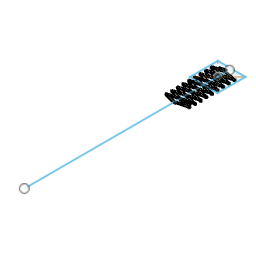
Scissor Cable Management_ (Autodesk Fusion 360 design; units mm, degrees)
Autodesk Fusion 360 part; units mm, degrees
sketch "Sketch1" plane through (0, 0, 0) normal (0, 1, 0) x (1, 0, 0) in component "Bottom"
  line L0 (0, 0) -> (0, 9) construction
  line L1 (0, 0) -> (54.8156, 4.5) construction
  line L2 (54.8156, 4.5) -> (0, 9) construction
  line L3 (0, 4.5) -> (54.8156, 4.5) construction
  line L4 (0, 9) -> (-54.8156, 13.5) construction
  line L5 (0, 0) -> (-54.8156, -4.5) construction
  line L6 (-55.1429, 9.5134) -> (54.4883, 0.5134)
  arc A0 (54.4883, 0.5134) -> (55.1429, 8.4866) centre (54.8156, 4.5) ccw
  line L7 (55.1429, 8.4866) -> (-54.4883, 17.4866)
  arc A1 (-54.4883, 17.4866) -> (-55.1429, 9.5134) centre (-54.8156, 13.5) ccw
  line L8 (-54.8156, 13.5) -> (54.8156, 4.5) construction
  line L9 (54.4883, 8.4866) -> (-55.1429, -0.5134)
  arc A2 (-55.1429, -0.5134) -> (-54.4883, -8.4866) centre (-54.8156, -4.5) ccw
  line L10 (-54.4883, -8.4866) -> (55.1429, 0.5134)
  arc A3 (55.1429, 0.5134) -> (54.4883, 8.4866) centre (54.8156, 4.5) ccw
  line L11 (54.8156, 4.5) -> (-54.8156, -4.5) construction
  circle A4 centre (-54.8156, -4.5) radius 1.6
  circle A5 centre (54.8156, 4.5) radius 1.6
  circle A6 centre (-54.8156, 13.5) radius 1.6
  circle A7 centre (0, 9) radius 1.6
  circle A8 centre (0, 0) radius 1.6
  circle A9 centre (0, 9) radius 4.5 construction
  circle A10 centre (0, 0) radius 4.5 construction
  point P0 (0, 4.5)
  dimension "d5" = 55
  dimension "d8" = 55
  dimension "d10" = 55
  dimension "d11" = 8
  dimension "d12" = 8
  dimension "d13" = 3.2
  dimension "d14" = 3.2
  dimension "d15" = 3.2
  dimension "d16" = 3.2
  dimension "d17" = 3.2
  dimension "d18" = 9
  dimension "d19" = 9
  constraint coincident L0.start L1.start
  constraint vertical L0
  constraint midpoint L0 P0
  constraint coincident P0 L3.start
  constraint horizontal L3
  constraint parallel L2 L4
  constraint parallel L1 L5
  constraint tangent L6 A0
  constraint tangent A0 L7
  constraint parallel L6 L7
  constraint tangent L7 A1
  constraint tangent L6 A1
  constraint coincident L1.end L2.start
  constraint parallel L2 L8
  constraint coincident L4.end A1.centre
  constraint tangent L9 A2
  constraint tangent A2 L10
  constraint parallel L9 L10
  constraint tangent L10 A3
  constraint tangent L9 A3
  constraint coincident L5.end A2.centre
  constraint parallel L5 L11
  constraint concentric A2 A4
  constraint concentric A3 A5
  constraint concentric A1 A6
  constraint coincident L0.end L2.end
  constraint concentric A7 A9
  constraint tangent A9 A10
  measures "d5" distance of L0.start L1.end
  measures "d8" distance of L0.end L4.end
  measures "d10" distance of L0.start L5.end
  measures "d11" diameter of A0
  measures "d12" diameter of A2
  measures "d13" diameter of A4
  measures "d14" diameter of A5
  measures "d15" diameter of A6
  measures "d16" diameter of A7
  measures "d17" diameter of A8
  measures "d18" diameter of A9
  measures "d19" diameter of A10
extrude "Extrude1" add sketch "Sketch1" along normal blind 3 contours L6 L7 A1 L9 A3 | L6 A0 L9 A3 makes body 1 in component "1"
extrude "Extrude1'" add sketch "Sketch1" against normal blind 3 separate body contours L6 A0 L9 A3 | L6 A0 L9 A2 L10 makes body 2 in component "2"
pattern_linear "00000000-0000-0000-0000-000000000000" [suppressed] in component "Bottom"
sketch "Sketch1 (2)" plane through (0, 0, 0) normal (0, 1, 0) x (1, 0, 0) in component "Top"
  line L0 (0, 0) -> (0, 9) construction
  line L1 (0, 0) -> (54.8156, 4.5) construction
  line L2 (54.8156, 4.5) -> (0, 9) construction
  line L3 (0, 4.5) -> (54.8156, 4.5) construction
  line L4 (0, 9) -> (-54.8156, 13.5) construction
  line L5 (0, 0) -> (-54.8156, -4.5) construction
  line L6 (-55.1429, 9.5134) -> (54.4883, 0.5134)
  arc A0 (54.4883, 0.5134) -> (55.1429, 8.4866) centre (54.8156, 4.5) ccw
  line L7 (55.1429, 8.4866) -> (-54.4883, 17.4866)
  arc A1 (-54.4883, 17.4866) -> (-55.1429, 9.5134) centre (-54.8156, 13.5) ccw
  line L8 (-54.8156, 13.5) -> (54.8156, 4.5) construction
  line L9 (54.4883, 8.4866) -> (-55.1429, -0.5134)
  arc A2 (-55.1429, -0.5134) -> (-54.4883, -8.4866) centre (-54.8156, -4.5) ccw
  line L10 (-54.4883, -8.4866) -> (55.1429, 0.5134)
  arc A3 (55.1429, 0.5134) -> (54.4883, 8.4866) centre (54.8156, 4.5) ccw
  line L11 (54.8156, 4.5) -> (-54.8156, -4.5) construction
  circle A4 centre (-54.8156, -4.5) radius 2.15
  circle A5 centre (54.8156, 4.5) radius 2.15
  circle A6 centre (-54.8156, 13.5) radius 2.15
  circle A7 centre (0, 9) radius 2.15
  circle A8 centre (0, 0) radius 2.15
  circle A9 centre (0, 9) radius 4.5 construction
  circle A10 centre (0, 0) radius 4.5 construction
  point P0 (0, 4.5)
  dimension "d5_1" = 55
  dimension "d8_1" = 55
  dimension "d10_1" = 55
  dimension "d11_1" = 8
  dimension "d12_1" = 8
  dimension "d13_1" = 4.3
  dimension "d14_1" = 4.3
  dimension "d15_1" = 4.3
  dimension "d16_1" = 4.3
  dimension "d17_1" = 4.3
  dimension "d18_1" = 9
  dimension "d19_1" = 9
  constraint coincident L0.start L1.start
  constraint vertical L0
  constraint midpoint L0 P0
  constraint coincident P0 L3.start
  constraint horizontal L3
  constraint parallel L2 L4
  constraint parallel L1 L5
  constraint tangent L6 A0
  constraint tangent A0 L7
  constraint parallel L6 L7
  constraint tangent L7 A1
  constraint tangent L6 A1
  constraint coincident L1.end L2.start
  constraint parallel L2 L8
  constraint coincident L4.end A1.centre
  constraint tangent L9 A2
  constraint tangent A2 L10
  constraint parallel L9 L10
  constraint tangent L10 A3
  constraint tangent L9 A3
  constraint coincident L5.end A2.centre
  constraint parallel L5 L11
  constraint concentric A2 A4
  constraint concentric A3 A5
  constraint concentric A1 A6
  constraint coincident L0.end L2.end
  constraint concentric A7 A9
  constraint tangent A9 A10
  measures "d5_1" distance of L0.start L1.end
  measures "d8_1" distance of L0.end L4.end
  measures "d10_1" distance of L0.start L5.end
  measures "d11_1" diameter of A0
  measures "d12_1" diameter of A2
  measures "d13_1" diameter of A4
  measures "d14_1" diameter of A5
  measures "d15_1" diameter of A6
  measures "d16_1" diameter of A7
  measures "d17_1" diameter of A8
  measures "d18_1" diameter of A9
  measures "d19_1" diameter of A10
extrude "Extrude1''" add sketch "Sketch1 (2)" along normal blind 3 separate body contours L6 L7 A1 L9 A3 | L6 A0 L9 A3 makes body 3 in component "1 (1)"
extrude "Extrude1'''" add sketch "Sketch1 (2)" against normal blind 3 separate body contours L6 A0 L9 A3 | L6 A0 L9 A2 L10 makes body 4 in component "2 (1)"
pattern_linear "R-Pattern1" [suppressed] in component "Top"
sketch "Sketch15" plane through (0, 0, 0) normal (0, 1, 0) x (1, 0, 0)
  line L0 (65, -95.4189) -> (-65, -95.4189)
  line L1 (-65, -95.4189) -> (-65, 35.4189)
  line L2 (-65, 35.4189) -> (65, 35.4189)
  line L3 (65, 35.4189) -> (65, -95.4189)
  line L4 (65, -95.4189) -> (-65, 35.4189) construction
  line L5 (-65, -95.4189) -> (65, 35.4189) construction
  point P0 (0, -30)
  dimension "d422" = 130
  constraint horizontal L0
  constraint perpendicular L0 L1
  constraint parallel L0 L2
  constraint parallel L1 L3
  constraint coincident L4 P0
  constraint coincident L5 P0
  measures "d422" distance of L1.end L2.end
sketch "Sketch1 (3)" plane through (0, -3, 0) normal (0, -1, 0) x (1, 0, 0) in component "Adapter"
  circle A0 centre (-54.8156, -4.5) radius 1.6
  circle A1 centre (0, -9) radius 1.6
  circle A2 centre (54.8156, -13.5) radius 1.6
  arc A3 (-54.4883, -0.5134) -> (-55.1429, -8.4866) centre (-54.8156, -4.5) ccw
  line L0 (-55.1429, -8.4866) -> (54.4883, -17.4866)
  arc A4 (54.4883, -17.4866) -> (55.1429, -9.5134) centre (54.8156, -13.5) ccw
  line L1 (55.1429, -9.5134) -> (-54.4883, -0.5134)
  circle A5 centre (0, -9) radius 1.6
  line L2 (9.1446, -15.4098) -> (-9.1446, -15.4098)
  line L3 (-9.1446, -15.4098) -> (-9.1446, -2.5902)
  line L4 (-9.1446, -2.5902) -> (9.1446, -2.5902)
  line L5 (9.1446, -2.5902) -> (9.1446, -15.4098)
  line L6 (9.1446, -15.4098) -> (-9.1446, -2.5902) construction
  line L7 (-9.1446, -15.4098) -> (9.1446, -2.5902) construction
  point P0 (0, -9)
  constraint horizontal L2
  constraint perpendicular L2 L3
  constraint parallel L2 L4
  constraint parallel L3 L5
  constraint coincident L6 P0
  constraint coincident L7 P0
  constraint coincident P0 A1.centre
extrude "Extrude1''''" add sketch "Sketch1 (3)" along normal blind 4 separate body contours L1 L3 L4 L5 | L0 L1 L3 L5 | L0 L2 L3 L5 makes body 5 in component "Adapter"
sketch "Sketch4" plane through (0, 0, 0) normal (0, 1, 0) x (1, 0, 0)
  line L0 (0, 25) -> (0, -935)
  dimension "d193" = 960
  constraint vertical L0
  measures "d193" distance of L0.start L0.end
sketch "Sketch3" plane through (0, 3, 0) normal (0, 1, 0) x (-1, 0, 0) in component "Top"
  circle A0 centre (0, -9) radius 2.15
  circle A1 centre (54.2857, -0.1646) radius 2.15
  circle A2 centre (-54.2857, -17.8354) radius 2.15
  arc A3 (54.9283, -4.1127) -> (53.6431, 3.7834) centre (54.2857, -0.1646) ccw
  line L0 (53.6431, 3.7834) -> (-54.9283, -13.8873)
  arc A4 (-54.9283, -13.8873) -> (-53.6431, -21.7834) centre (-54.2857, -17.8354) ccw
  line L1 (-53.6431, -21.7834) -> (54.9283, -4.1127)
  line L2 (-54.2857, -17.8354) -> (0, -9) construction
  line L3 (0, -9) -> (54.2857, -0.1646) construction
  line L4 (-27.1428, -13.4177) -> (-27.7854, -9.4696)
  line L5 (-27.1428, -13.4177) -> (-26.5003, -17.3657) construction
  line L6 (0, -9) -> (-0.5388, -5.6896) construction
  line L7 (-24.1818, -12.9358) -> (-24.8244, -8.9877)
  line L8 (-24.1818, -12.9358) -> (-23.5392, -16.8838)
  line L9 (-30.1039, -13.8996) -> (-30.7465, -9.9516)
  line L10 (-30.1039, -13.8996) -> (-29.4613, -17.8477)
  line L11 (24.1818, -5.0642) -> (23.5392, -1.1162)
  line L12 (24.1818, -5.0642) -> (24.8244, -9.0123)
  line L13 (30.1039, -4.1004) -> (29.4613, -0.1523)
  line L14 (30.1039, -4.1004) -> (30.7465, -8.0484)
  dimension "d243" = 3
  dimension "d244" = -3
  constraint coincident A2.centre A4.centre
  constraint coincident A0.centre L2.end
  constraint coincident A1.centre A3.centre
  constraint midpoint L2 L4.start
  constraint coincident L0 L4.end
  constraint perpendicular L0 L4
  constraint coincident L1 L5.end
  constraint perpendicular L1 L5
  constraint perpendicular L3 L6
  constraint symmetric L6 L7.start L11.start
  constraint symmetric L6 L7.end L11.end
  constraint symmetric L6 L8.end L12.end
  constraint symmetric L6 L9.start L13.start
  constraint symmetric L6 L9.end L13.end
  constraint symmetric L6 L10.end L14.end
extrude "Extrude4" add sketch "Sketch3" along normal blind 6 contours L0 L1 L11 L12 L13 L14 | L0 L1 L7 L8 L9 L10 sketch seen with x (-0.97056, 0, -0.24086) y (0, 1, 0) z (0.24086, 0, -0.97056) at (2.1677, 0, -17.735) bodies 3 in component "1 (1)"
sketch "Sketch1 (4)" plane through (29.6638, 0, 2.4352) normal (0.996647, 0, 0.081818) x (0.081818, 0, -0.996647) in component "1 (1)"
  line L0 (4.9698, 3) -> (12.9698, 3)
  line L1 (12.9698, 3) -> (12.9698, 9)
  line L2 (12.9698, 9) -> (4.9698, 9)
  line L3 (4.9698, 9) -> (4.9698, 3)
  line L4 (8.9698, 9) -> (8.9698, 3) construction
  circle A0 centre (8.9698, 5) radius 4
  circle A1 centre (8.9698, 5) radius 2
  dimension "d248" = 8
  dimension "d249" = 4
  constraint midpoint L2 L4.start
  constraint midpoint L0 L4.end
  constraint coincident L4.start A0
  constraint concentric A0 A1
  measures "d248" diameter of A0
  measures "d249" diameter of A1
extrude "Extrude5" cut sketch "Sketch1 (4)" against normal blind 69 contours A1 | L2 L3 A0 | L1 L2 A0 bodies 3 in component "1 (1)"
sketch "Sketch2" plane through (0, 3, 2.4175) normal (0, 1, 0) x (-1, 0, 0) in component "Bottom"
  circle A0 centre (-54.2857, -2.5821) radius 1.6
  circle A1 centre (0, 6.2532) radius 1.6
  circle A2 centre (54.2857, 15.0886) radius 1.6
  arc A3 (-54.9283, 1.3659) -> (-53.6431, -6.5302) centre (-54.2857, -2.5821) ccw
  line L0 (-53.6431, -6.5302) -> (54.9283, 11.1406)
  arc A4 (54.9283, 11.1406) -> (53.6431, 19.0367) centre (54.2857, 15.0886) ccw
  line L1 (53.6431, 19.0367) -> (-54.9283, 1.3659)
  line L2 (0, 6.2532) -> (-54.2857, -2.5821) construction
  line L3 (0, 6.2532) -> (54.2857, 15.0886) construction
  line L4 (-27.1428, 1.8355) -> (-27.7854, 5.7836)
  line L5 (-27.1428, 1.8355) -> (-26.5003, -2.1125) construction
  line L6 (-24.1818, 2.3175) -> (-24.8244, 6.2655)
  line L7 (-24.1818, 2.3175) -> (-23.5392, -1.6306)
  line L8 (-30.1039, 1.3536) -> (-30.7465, 5.3017)
  line L9 (-30.1039, 1.3536) -> (-29.4613, -2.5944)
  line L10 (0, 6.2532) -> (-0.257, 7.8325) construction
  line L11 (24.1818, 10.189) -> (23.5392, 14.137)
  line L12 (30.1039, 11.1528) -> (29.4613, 15.1009)
  line L13 (30.1039, 11.1528) -> (30.7465, 7.2048)
  line L14 (24.1818, 10.189) -> (24.8244, 6.2409)
  dimension "d252" = 3
  dimension "d253" = -3
  constraint coincident A1.centre L2.start
  constraint coincident A0.centre A3.centre
  constraint coincident A2.centre A4.centre
  constraint midpoint L2 L4.start
  constraint coincident L1 L4.end
  constraint perpendicular L1 L4
  constraint coincident L0 L5.end
  constraint perpendicular L0 L5
  constraint coincident A1 L10.end
  constraint perpendicular L3 L10
  constraint symmetric L6.start L10 L11.start
  constraint symmetric L6.end L10 L11.end
  constraint symmetric L7.end L10 L14.end
  constraint symmetric L8.start L10 L12.start
  constraint symmetric L8.end L10 L12.end
  constraint symmetric L9.end L10 L13.end
extrude "Extrude2" add sketch "Sketch2" along normal blind 6 contours L0 L1 L6 L7 L8 L9 | L0 L1 L11 L12 L13 L14 sketch seen with x (0.97056, 0, -0.24086) y (0, -1, 0) z (-0.24086, 0, -0.97056) at (2.0884, 0, 8.4155) bodies 2 in component "2"
sketch "Sketch1 (5)" plane through (-30.3977, 0, 2.4955) normal (-0.996647, 0, 0.081818) x (0.081818, 0, 0.996647) in component "2"
  line L0 (4, -3) -> (-4, -3)
  line L1 (-4, -3) -> (-4, -9)
  line L2 (-4, -9) -> (4, -9)
  line L3 (4, -9) -> (4, -3)
  line L4 (0, -9) -> (0, -1) construction
  circle A0 centre (0, -5) radius 4
  circle A1 centre (0, -5) radius 2
  dimension "d256" = 8
  dimension "d257" = 8
  dimension "d258" = 4
  constraint midpoint L2 L4.start
  constraint perpendicular L2 L4
  constraint midpoint L4 A0.centre
  constraint concentric A0 A1
  measures "d256" distance of L4.start L4.end
  measures "d257" diameter of A0
  measures "d258" diameter of A1
extrude "Extrude3" cut sketch "Sketch1 (5)" against normal blind 68 contours A1 | L2 L3 A0 | L1 L2 A0 bodies 2 in component "2"
extrude "Extrude1'''''" add sketch "Sketch1" against normal blind 3 separate body contours L6 L7 A1 L9 A3 | L6 A0 L9 A3 makes body 6 in component "Terminator"
sketch "Sketch1 (6)" plane through (0, 0, 0) normal (0, 1, 0) x (-1, 0, 0) in component "Terminator"
  circle A0 centre (0, -9) radius 1.6
  circle A1 centre (-54.8156, -4.5) radius 1.6
  circle A2 centre (54.8156, -13.5) radius 1.6
  arc A3 (-54.4883, -0.5134) -> (-55.1429, -8.4866) centre (-54.8156, -4.5) ccw
  line L0 (-55.1429, -8.4866) -> (54.4883, -17.4866)
  arc A4 (54.4883, -17.4866) -> (55.1429, -9.5134) centre (54.8156, -13.5) ccw
  line L1 (55.1429, -9.5134) -> (-54.4883, -0.5134)
  line L2 (-55.1586, -8.6783) -> (-0.343, -13.1783)
  arc A5 (-0.343, -13.1783) -> (0.343, -4.8217) centre (0, -9) ccw
  line L3 (0.343, -4.8217) -> (-54.4726, -0.3217)
  arc A6 (-54.4726, -0.3217) -> (-55.1586, -8.6783) centre (-54.8156, -4.5) ccw
  line L4 (-54.8156, -4.5) -> (0, -9) construction
  constraint tangent L2 A5
  constraint tangent A5 L3
  constraint parallel L2 L3
  constraint tangent L3 A6
  constraint tangent L2 A6
  constraint coincident A0.centre A5.centre
  constraint parallel L0 L4
  constraint coincident A1.centre A3.centre
extrude "Extrude2'" cut sketch "Sketch1 (6)" against normal blind 3 contours L0 A4 L1 A5 bodies 6 in component "Terminator"
extrude "Extrude1''''''" add sketch "Sketch1" along normal blind 3 separate body contours L6 L7 A1 L9 A3 | L6 A0 L9 A3 makes body 7 in component "Terminator (1)"
sketch "Sketch1 (7)" plane through (0, 3, 0) normal (0, 1, 0) x (-1, 0, 0) in component "Terminator (1)"
  circle A0 centre (0, -9) radius 1.6
  circle A1 centre (-54.8156, -4.5) radius 1.6
  circle A2 centre (54.8156, -13.5) radius 1.6
  arc A3 (-54.4883, -0.5134) -> (-55.1429, -8.4866) centre (-54.8156, -4.5) ccw
  line L0 (-55.1429, -8.4866) -> (54.4883, -17.4866)
  arc A4 (54.4883, -17.4866) -> (55.1429, -9.5134) centre (54.8156, -13.5) ccw
  line L1 (55.1429, -9.5134) -> (-54.4883, -0.5134)
  line L2 (-0.343, -13.1783) -> (54.4726, -17.6783)
  arc A5 (54.4726, -17.6783) -> (55.1586, -9.3217) centre (54.8156, -13.5) ccw
  line L3 (55.1586, -9.3217) -> (0.343, -4.8217)
  arc A6 (0.343, -4.8217) -> (-0.343, -13.1783) centre (0, -9) ccw
  line L4 (0, -9) -> (54.8156, -13.5) construction
  constraint tangent L2 A5
  constraint tangent A5 L3
  constraint parallel L2 L3
  constraint tangent L3 A6
  constraint tangent L2 A6
  constraint coincident A2.centre A4.centre
  constraint coincident A0.centre A6.centre
extrude "Extrude2''" cut sketch "Sketch1 (7)" against normal blind 3 contours A3 L0 L1 A6 bodies 7 in component "Terminator (1)"
sketch "Sketch2 (2)" plane through (0, 3, 0) normal (0, 1, 0) x (-1, 0, 0) in component "Terminator (1)"
  arc A0 (-0.924, -4.9107) -> (-1.5786, -12.8839) centre (0, -9) ccw
  line L0 (-1.5786, -12.8839) -> (54.4883, -17.4866)
  arc A1 (54.4883, -17.4866) -> (55.1429, -9.5134) centre (54.8156, -13.5) ccw
  line L1 (55.1429, -9.5134) -> (-0.924, -4.9107)
  circle A2 centre (0, -9) radius 1.6
  circle A3 centre (54.8156, -13.5) radius 1.6
  line L2 (0, -9) -> (54.8156, -13.5) construction
  line L3 (27.4078, -11.25) -> (27.1094, -7.212)
  line L4 (27.4078, -11.25) -> (26.4549, -15.1852) construction
  line L5 (30.4343, -11.4985) -> (30.1013, -6.991)
  line L6 (30.4343, -11.4985) -> (29.3706, -15.8913)
  line L7 (24.3813, -11.0015) -> (24.1176, -7.4331)
  line L8 (24.3813, -11.0015) -> (23.5392, -14.4792)
  dimension "d289" = 3
  dimension "d290" = -3
  constraint coincident A0.centre A2.centre
  constraint coincident A1.centre A3.centre
  constraint midpoint L2 L3.start
  constraint midpoint L1 L3.end
  constraint midpoint L0 L4.end
extrude "Extrude3'" add sketch "Sketch2 (2)" along normal blind 6 contours A0 L0 L1 L5 L6 | A2 bodies 7 in component "Terminator (1)"
sketch "Sketch3 (2)" plane through (-31.3787, 0, -7.5983) normal (-0.971911, 0, -0.235348) x (-0.235348, 0, 0.971911) in component "Terminator (1)"
  line L0 (-4.0128, 3) -> (-0.1585, 3)
  line L1 (-0.1585, 3) -> (-0.1585, 9)
  line L2 (-0.1585, 9) -> (-4.0128, 9)
  line L3 (-8.0618, 9) -> (-8.0618, 3)
  line L4 (-2.0857, 9) -> (-2.0857, 1) construction
  circle A0 centre (-2.0857, 5) radius 1.9272
  circle A1 centre (-2.0857, 5) radius 2
  line L5 (-4.0128, 9) -> (-4.0128, 3)
  line L6 (-8.0618, 3) -> (-4.0128, 3)
  line L7 (-4.0128, 3) -> (-4.0128, 9)
  line L8 (-4.0128, 9) -> (-8.0618, 9)
  dimension "d293" = 8
  dimension "d294" = 4
  constraint midpoint L2 L4.start
  constraint perpendicular L2 L4
  constraint midpoint L4 A0.centre
  constraint tangent L1 A0
  constraint concentric A0 A1
  measures "d293" distance of L4.start L4.end
  measures "d294" diameter of A1
extrude "Extrude4'" cut sketch "Sketch3 (2)" against normal blind 10 bodies 7 in component "Terminator (1)"
component "Bottom" placed x (1, 0, 0) y (0, 1, 0) z (0, 0, 1) at (0, 0, 0)
component "Top" placed x (1, 0, 0) y (0, 1, 0) z (0, 0, 1) at (0, 0, 0)
component "Adapter" placed x (1, 0, 0) y (0, 1, 0) z (0, 0, 1) at (0, 0, 0)
component "2" placed x (0.940553, 0, -0.339647) y (0, -1, 0) z (-0.339647, 0, -0.940553) at (0.463, 0, 17.9383) in component "Bottom"
component "1" placed x (0.951669, 0, 0.307127) y (0, -1, 0) z (0.307127, 0, -0.951669) at (3.6901, 0, 36.3116) in component "Bottom"
component "2" placed x (0.940553, 0, -0.339647) y (0, -1, 0) z (-0.339647, 0, -0.940553) at (1.3889, 0, 71.8149) in component "Bottom"
component "1" placed x (0.951669, 0, 0.307127) y (0, -1, 0) z (0.307127, 0, -0.951669) at (4.616, 0, 90.1882) in component "Bottom"
component "2" placed x (0.940553, 0, -0.339647) y (0, -1, 0) z (-0.339647, 0, -0.940553) at (2.3149, 0, 125.6916) in component "Bottom"
component "1" placed x (0.951669, 0, 0.307127) y (0, -1, 0) z (0.307127, 0, -0.951669) at (5.542, 0, 144.0648) in component "Bottom"
component "2" placed x (0.940553, 0, -0.339647) y (0, -1, 0) z (-0.339647, 0, -0.940553) at (3.2408, 0, 179.5682) in component "Bottom"
component "1" placed x (0.951669, 0, 0.307127) y (0, -1, 0) z (0.307127, 0, -0.951669) at (6.4679, 0, 197.9415) in component "Bottom"
component "Terminator" placed x (0.989016, 0, 0.147809) y (0, 1, 0) z (-0.147809, 0, 0.989016) at (-1.3303, 0, -0.0989) in component "Bottom"
component "Terminator (1)" placed x (0.940553, 0, -0.339647) y (0, 1, 0) z (0.339647, 0, 0.940553) at (60.309, 0, 227.5243) in component "Bottom"
component "2 (1)" placed x (-0.951669, 0, -0.307127) y (0, 1, 0) z (0.307127, 0, -0.951669) at (0.463, 0, 17.9383) in component "Top"
component "1 (1)" placed x (-0.940553, 0, 0.339647) y (0, 1, 0) z (-0.339647, 0, -0.940553) at (-2.1309, 0, 36.4116) in component "Top"
component "2 (1)" placed x (-0.951669, 0, -0.307127) y (0, 1, 0) z (0.307127, 0, -0.951669) at (1.3889, 0, 71.8149) in component "Top"
component "1 (1)" placed x (-0.940553, 0, 0.339647) y (0, 1, 0) z (-0.339647, 0, -0.940553) at (-1.2049, 0, 90.2883) in component "Top"
component "2 (1)" placed x (-0.951669, 0, -0.307127) y (0, 1, 0) z (0.307127, 0, -0.951669) at (2.3149, 0, 125.6916) in component "Top"
component "1 (1)" placed x (-0.940553, 0, 0.339647) y (0, 1, 0) z (-0.339647, 0, -0.940553) at (-0.279, 0, 144.1649) in component "Top"
component "2 (1)" placed x (-0.951669, 0, -0.307127) y (0, 1, 0) z (0.307127, 0, -0.951669) at (3.2408, 0, 179.5682) in component "Top"
component "1 (1)" placed x (-0.940553, 0, 0.339647) y (0, 1, 0) z (-0.339647, 0, -0.940553) at (0.6469, 0, 198.0415) in component "Top"
component "Terminator (1)" placed x (0.940553, 0, -0.339647) y (0, 1, 0) z (0.339647, 0, 0.940553) at (3.0568, 0, -0.535) in component "Top"
component "Terminator" placed x (0.989016, 0, 0.147809) y (0, 1, 0) z (-0.147809, 0, 0.989016) at (-50.7119, 0, 229.7931) in component "Top"
hidden bodies 5
equation "pivotSpacing = 7.5 mm"
equation "segLength = 110 mm"
equation "numberPivots = 5"
equation "d5 = segLength / 2"
equation "segThickness = 3 mm"
equation "segWidth = 8 mm"
equation "d8 = segLength / 2"
equation "d10 = segLength / 2"
equation "d11 = segWidth"
equation "d12 = segWidth"
equation "d22 = segThickness"
equation "d34 = numberPivots"
equation "d193 = ( 240 * 4 ) * 1 mm"
equation "d5_1 = segLength / 2"
equation "d8_1 = segLength / 2"
equation "d10_1 = segLength / 2"
equation "d11_1 = segWidth"
equation "d12_1 = segWidth"
equation "d22_1 = segThickness"
equation "d34_1 = numberPivots"
equation "d261 = -segThickness"
equation "d277 = segThickness"
